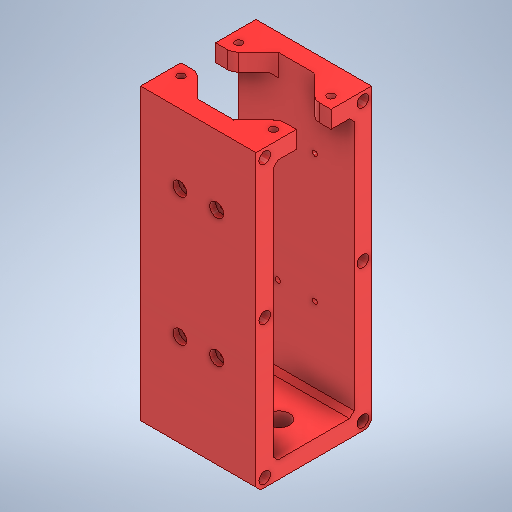
# Autodesk Inventor part: Main_Cover
Saved by Autodesk Inventor 2026.2 (Build 302298010, 298A)
## iProperties
Created: 2026-05-07
Part Number: Main_Cover
Material: Generic
Document SubType Name: Modeling
Designer: piete
Density: 1 g/cm^3
Appearance: Light Red
Author: piete
Autodesk Inventor part; units mm, degrees
ref_plane "YZ Plane" through (0, 0, 0) normal (1, 0, 0) x (0, 1, 0)
ref_plane "XZ Plane" through (0, 0, 0) normal (0, 1, 0) x (-1, 0, 0)
ref_plane "XY Plane" through (0, 0, 0) normal (0, 0, 1) x (1, 0, 0)
sketch "Sketch1" plane through (0, 0, 0) normal (0, 1, 0) x (-1, 0, 0)
  line L0 (25, 25) -> (-25, 25)
  line L1 (-25, 25) -> (-25, -25)
  line L2 (-25, -25) -> (25, -25)
  line L3 (25, -25) -> (25, 25)
  point P0 (0, 0)
  dimension "d0" = 50
  dimension "d1" = 50
  dimension "d2" = 25
  dimension "d3" = 25
  constraints: 8 end point, 2 parallel, 1 horizontal, 1 perpendicular
  measures "d0" distance of L2.end L0.start
  measures "d1" distance of L1.end L2.end
  measures "d2" distance from line of point (0, 0) L3
  measures "d3" distance from line of L2 point (0, 0)
extrude "Extrusion1" add sketch "Sketch1" along normal blind 7.5
sketch "Sketch2" plane through (0, 7.5, 0) normal (0, 1, 0) x (1, 0, 0)
  line L0 (-25, 25) -> (-25, -25) projected
  line L1 (25, -25) -> (25, 25) projected
  line L2 (-25, -25) -> (25, -25)
  line L3 (25, -25) -> (25, -17.5)
  line L4 (25, -17.5) -> (-25, -17.5)
  line L5 (-25, -17.5) -> (-25, -25)
  line L6 (-25, 25) -> (25, 25)
  line L7 (25, 25) -> (25, 17.5)
  line L8 (25, 17.5) -> (-25, 17.5)
  line L9 (-25, 17.5) -> (-25, 25)
  point P0 (0, 0)
  point P1 (-25, -17.5)
  point P2 (-25, 17.5)
  dimension "d6" = 7.5
  dimension "d7" = 7.5
  dimension "d8" = 25
  constraints: 16 end point, 4 parallel, 3 point on line, 2 horizontal, 2 perpendicular
  measures "d6" distance of L3.end L2.end
  measures "d7" distance of L6.end L7.end
  measures "d8" distance from line of point (0, 0) L6
extrude "Extrusion2" add sketch "Sketch2" along normal blind 120 contours L6 L1 L8 L0 | L4 L1 L2 L0
sketch "Sketch3" plane through (-25, 0, 25) normal (0, 0, 1) x (1, 0, 0)
  circle A0 centre (33, 97.5) radius 1.1
  circle A1 centre (33, 42) radius 1.1
  circle A2 centre (17, 42) radius 1.1
  circle A3 centre (17, 97.5) radius 1.1
  line L0 (50, 0) -> (50, 127.5) projected
  line L1 (0, 0) -> (0, 127.5) projected
  line L2 (0, 127.5) -> (50, 127.5) projected
  point P0 (25, 0)
  dimension "d11" = 2.2
  dimension "d12" = 2.2
  dimension "d13" = 2.2
  dimension "d14" = 2.2
  dimension "d15" = 55.5
  dimension "d17" = 55.5
  dimension "d18" = 17
  dimension "d19" = 17
  dimension "d20" = 17
  dimension "d21" = 17
  dimension "d22" = 30
  dimension "d23" = 30
  constraints: 4 centre point
  measures "d11" diameter of A0
  measures "d12" diameter of A1
  measures "d13" diameter of A2
  measures "d14" diameter of A3
  measures "d15" distance of A2.centre A3.centre
  measures "d17" distance of A0.centre A1.centre
  measures "d18" distance from line of L0 A0.centre
  measures "d19" distance from line of L0 A1.centre
  measures "d20" distance from line of L1 A3.centre
  measures "d21" distance from line of L1 A2.centre
  measures "d22" distance from line of L2 A3.centre
  measures "d23" distance from line of L2 A0.centre
extrude "Extrusion3" cut sketch "Sketch3" against normal through all
sketch "Sketch4" plane through (-25, 0, 25) normal (0, 0, 1) x (1, 0, 0)
  circle A0 centre (17, 97.5) radius 1.1 projected
  circle A1 centre (17, 97.5) radius 3
  circle A2 centre (33, 97.5) radius 1.1 projected
  circle A3 centre (33, 97.5) radius 3
  circle A4 centre (17, 42) radius 1.1 projected
  circle A5 centre (17, 42) radius 3
  circle A6 centre (33, 42) radius 1.1 projected
  circle A7 centre (33, 42) radius 3
  point P0 (25, 0)
  dimension "d26" = 6
  dimension "d27" = 6
  dimension "d28" = 6
  dimension "d29" = 6
  constraints: 4 centre point, 4 coincident
  measures "d26" diameter of A1
  measures "d27" diameter of A3
  measures "d28" diameter of A5
  measures "d29" diameter of A7
extrude "Extrusion4" cut sketch "Sketch4" against normal blind 2.5 contours A1 | A2 | A3 | A5 | A7
sketch "Sketch5" plane through (0, 127.5, 0) normal (0, 1, 0) x (1, 0, 0)
  circle A0 centre (-20, -12.5) radius 1.6
  circle A1 centre (-20, 12.5) radius 1.6
  line L0 (-25, 17.5) -> (-25, -17.5) projected
  line L1 (-25, 17.5) -> (25, 17.5) projected
  line L2 (25, -17.5) -> (-25, -17.5) projected
  circle A2 centre (-20, -12.5) radius 5
  circle A3 centre (-20, 12.5) radius 5
  line L3 (-25, 17.5) -> (-25, 7.5)
  line L4 (-25, 7.5) -> (-20, 7.5)
  line L5 (25, 17.5) -> (-25, 17.5) projected
  line L6 (-7.9289, 17.5) -> (-16.4645, 8.9645)
  line L7 (-7.9289, 17.5) -> (9.8712, 17.5) construction
  line L8 (-25, 25) -> (-25, 17.5) projected
  line L9 (-25, 17.5) -> (-7.9289, 17.5)
  line L10 (-25, -17.5) -> (-25, -25) projected
  line L11 (-25, -17.5) -> (-25, -7.5)
  line L12 (-25, 25) -> (-25, -25) projected
  line L13 (-25, -7.5) -> (-20, -7.5)
  line L14 (-7.9289, -17.5) -> (-16.4645, -8.9645)
  line L15 (-7.9289, -17.5) -> (7.3912, -17.5) construction
  line L16 (-7.9289, -17.5) -> (-25, -17.5)
  point P0 (0, 0)
  dimension "d32" = 3.2
  dimension "d33" = 3.2
  dimension "d34" = 5
  dimension "d35" = 5
  dimension "d36" = 5
  dimension "d37" = 5
  dimension "d38" = 10
  dimension "d39" = 10
  dimension "d40" = 10
  dimension "d41" = 135
  dimension "d42" = 10
  dimension "d43" = 5
  dimension "d44" = 135
  constraints: 20 end point, 4 centre point, 4 point on circle, 4 point on line, 3 horizontal, 2 coincident, 2 tangent, 1 collinear, 1 perpendicular
  measures "d32" diameter of A0
  measures "d33" diameter of A1
  measures "d34" distance from line of L0 A1.centre
  measures "d35" distance from line of L1 A1.centre
  measures "d36" distance from line of L0 A0.centre
  measures "d37" distance from line of L2 A0.centre
  measures "d38" diameter of A2
  measures "d39" diameter of A3
  measures "d40" distance of L0.start L3.end
  measures "d41" angle of L6 L7
  measures "d42" distance of L0.end L11.end
  measures "d43" distance of L11.end L13.end
  measures "d44" angle of L15 L14
extrude "Extrusion5" add sketch "Sketch5" against normal blind 7.5
mirror "Mirror1" about plane through (0, 0, 0) normal (1, 0, 0) of "Extrusion5"
sketch "Sketch6" plane through (0, 0, 0) normal (0, -1, 0) x (1, 0, 0)
  circle A0 centre (-10, 0) radius 4.5
  circle A1 centre (10, 0) radius 4.5
  line L0 (0, 35) -> (0, -35) projected
  line L1 (25, 25) -> (25, -25) projected
  circle A2 centre (0, 0) radius 1
  point P0 (25, 0)
  dimension "Festo_Clips" = 9
  dimension "d48" = 9
  dimension "d49" = 0
  dimension "d50" = 10
  dimension "d51" = 10
  dimension "d52" = 0
  dimension "d77" = 2
  constraints: 3 centre point, 1 coincident, 1 midpoint
  measures "Festo_Clips" diameter of A0
  measures "d48" diameter of A1
  measures "d49" vertical distance of A1.centre A0.centre
  measures "d50" distance from line of L0 A0.centre
  measures "d51" distance from line of L0 A1.centre
  measures "d52" vertical distance of point (25, 0) A0.centre
  measures "d77" diameter of A2
extrude "Extrusion6" cut sketch "Sketch6" against normal blind 7.5
sketch "Sketch7" plane through (-25, 0, -25) normal (-1, 0, 0) x (0, 0, 1)
  circle A0 centre (3.75, 3.75) radius 1.5
  circle A1 centre (3.75, 63.75) radius 1.5
  circle A2 centre (3.75, 123.75) radius 1.5
  line L0 (0, 0) -> (0, 127.5) projected
  line L1 (0, 127.5) -> (17.5, 127.5) projected
  line L2 (0, 0) -> (50, 0) projected
  point P0 (25, 0)
  dimension "d55" = 3
  dimension "d56" = 3
  dimension "d57" = 3
  dimension "d58" = 3.75
  dimension "d59" = 3.75
  dimension "d60" = 3.75
  dimension "d61" = 3.75
  dimension "d62" = 3.75
  dimension "d63" = 63.75
  constraints: 3 centre point
  measures "d55" diameter of A0
  measures "d56" diameter of A1
  measures "d57" diameter of A2
  measures "d58" distance from line of L0 A2.centre
  measures "d59" distance from line of L1 A2.centre
  measures "d60" distance from line of L0 A1.centre
  measures "d61" distance from line of L0 A0.centre
  measures "d62" distance from line of L2 A0.centre
  measures "d63" distance from line of L2 A1.centre
extrude "Extrusion7" cut sketch "Sketch7" against normal blind 4
mirror "Mirror2" about plane through (0, 0, 0) normal (1, 0, 0) of "Extrusion7"
mirror "Mirror3" about plane through (0, 0, 0) normal (0, 0, 1) of "Extrusion7", "Mirror2"
sketch "Sketch8" plane through (25, 0, 25) normal (1, 0, 0) x (0, 0, -1)
  circle A0 centre (46.25, 3.75) radius 1.5 projected
  circle A1 centre (46.25, 3.75) radius 2.5
  circle A2 centre (3.75, 3.75) radius 1.5 projected
  circle A3 centre (3.75, 3.75) radius 2.5
  circle A4 centre (3.75, 63.75) radius 1.5 projected
  circle A5 centre (3.75, 63.75) radius 2.5
  circle A6 centre (46.25, 63.75) radius 1.5 projected
  circle A7 centre (46.25, 63.75) radius 2.5
  circle A8 centre (46.25, 123.75) radius 1.5 projected
  circle A9 centre (46.25, 123.75) radius 2.5
  circle A10 centre (3.75, 123.75) radius 1.5 projected
  circle A11 centre (3.75, 123.75) radius 2.5
  point P0 (25, 0)
  dimension "d66" = 5
  dimension "d67" = 5
  dimension "d68" = 5
  dimension "d69" = 5
  dimension "d70" = 5
  dimension "d71" = 5
  constraints: 6 centre point, 6 coincident
  measures "d66" diameter of A1
  measures "d67" diameter of A3
  measures "d68" diameter of A5
  measures "d69" diameter of A7
  measures "d70" diameter of A9
  measures "d71" diameter of A11
extrude "Extrusion8" cut sketch "Sketch8" against normal blind 5.1 contours A0 | A1 | A2 | A3 | A4 | A5 | A6 | A7 | A8 | A9 | A10 | A11
mirror "Mirror4" about plane through (0, 0, 0) normal (1, 0, 0) of "Extrusion8"
chamfer "Chamfer1" distance 2 angle 45 8 edges at (0, 0, 25) (0, 0, -25) (0, 7.5, -17.5) (0, 7.5, 17.5) (16.4645, 120, -17.5) (16.4645, 120, 17.5) (-16.4645, 120, -17.5) (-16.4645, 120, 17.5)
mirror "Mirror5" about plane through (0, 0, 0) normal (0, 0, 1) of "Extrusion4"
equation "\"d2\" = 0.5 * d1"
equation "\"d3\" = 0.5 * d0"
equation "\"d6\" = Thickness"
equation "\"d7\" = Thickness"
equation "\"d8\" = 0.5 * d1"
equation "\"d45\" = Thickness"
equation "\"d48\" = Festo_Clips"
equation "\"d53\" = Thickness"
equation "\"d58\" = 0.5 * Thickness"
equation "\"d59\" = 0.5 * Thickness"
equation "\"d60\" = 0.5 * Thickness"
equation "\"d61\" = 0.5 * Thickness"
equation "\"d62\" = 0.5 * Thickness"
equation "\"Thickness\" = 7.5"
body "Solid1"
